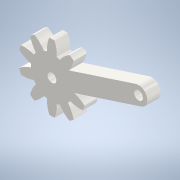
# Autodesk Inventor part: Spur Gear2
Saved by Autodesk Inventor 2021 (Build 250183000, 183)
## iProperties
CustomPartVersion: 1
Created: 2022-01-08
Part Number: Spur Gear2
Material: Steel
Document SubType Name: Modeling
Designer: Łukasz
Categories: <?xml version="1.0" encoding="UTF-16"?> <MemberInstance><Categories><FamilyTemplate><FamilyTemplateParameter ValueType="xs:double" Id="1" ObjectReferenceKey="da_z" ObjectType="kUserParameterObject"/><FamilyTemplateParameter ValueType="xs:double" Id="2" ObjectReferenceKey="da_b" ObjectType="kUserParameterObject"/><FamilyTemplateParameter ValueType="xs:double" Id="3" ObjectReferenceKey="da_beta" ObjectType="kUserParameterObject"/><FamilyTemplateParameter ValueType="xs:double" Id="4" ObjectReferenceKey="da_da" ObjectType="kUserParameterObject"/><FamilyTemplateParameter ValueType="xs:double" Id="5" ObjectReferenceKey="da_aw" ObjectType="kUserParameterObject"/><FamilyTemplateParameter ValueType="xs:string" Id="6" ObjectReferenceKey="EAIAABAAAACIAQAAAAAAAIAAAAAAAAAA" ObjectType="83910656" SubObjectId="SurfaceGeometry"/></FamilyTemplate><ParamToTemplateMap><ParamToTemplate CategoryParameter="//CategoryParameter[@InternalName='046C89C9-8512-4d59-83FE-43B91F4F132A']" TemplateParameter="1"/><ParamToTemplate CategoryParameter="//CategoryParameter[@InternalName='2552DF32-E462-4b46-AEBF-C6C7768E72AC']" TemplateParameter="2"/><ParamToTemplate CategoryParameter="//CategoryParameter[@InternalName='C9EE641D-15FC-4fae-A226-E94C4372FDD7']" TemplateParameter="3"/><ParamToTemplate><ParamToTemplate CategoryParameter="//CategoryParameter[@InternalName='00B6519A-459B-49c7-AD84-2E56D39A5744']" ConstantValue="0.035848"/></ParamToTemplate><ParamToTemplate><ParamToTemplate CategoryParameter="//CategoryParameter[@InternalName='04B31F0E-C7A6-4894-AA32-9629BEFACF47']" ConstantValue="1.000000"/></ParamToTemplate><ParamToTemplate><ParamToTemplate CategoryParameter="//CategoryParameter[@InternalName='43CBEC2E-7847-49e7-A936-2F7889FCB2D9']" ConstantValue="0.250000"/></ParamToTemplate><ParamToTemplate><ParamToTemplate CategoryParameter="//CategoryParameter[@InternalName='B1EFC894-105D-4ebd-86BF-FA20ED196853']" ConstantValue="0.302500"/></ParamToTemplate><ParamToTemplate><ParamToTemplate CategoryParameter="//CategoryParameter[@InternalName='51175063-3D10-4879-93E8-6246FE8B403D']" ConstantValue="2060000000.000000"/></ParamToTemplate><ParamToTemplate><ParamToTemplate CategoryParameter="//CategoryParameter[@InternalName='A3A52E27-4454-46a9-B0BD-C932399B70AF']" ConstantValue="0.300000"/></ParamToTemplate><ParamToTemplate><ParamToTemplate CategoryParameter="//CategoryParameter[@InternalName='91B76062-C214-41d9-B1B9-14D2AB99603D']" ConstantValue="0.250000"/></ParamToTemplate><ParamToTemplate><ParamToTemplate CategoryParameter="//CategoryParameter[@InternalName='374E806E-8B8A-4dda-A9AA-1039D6500AD2']" ConstantValue="4.000000"/></ParamToTemplate><ParamToTemplate><ParamToTemplate CategoryParameter="//CategoryParameter[@InternalName='2D373A89-B862-43d6-8D0B-0CBF12AB9F6C']" ConstantValue="0.349066"/></ParamToTemplate><ParamToTemplate CategoryParameter="//CategoryParameter[@InternalName='37777632-D6A2-4fac-9D53-DB8ACD95C989']" TemplateParameter="4"/><ParamToTemplate CategoryParameter="//CategoryParameter[@InternalName='FD1017F1-B727-4f7e-9707-0F86F1FF9423']" TemplateParameter="5"/><ParamToTemplate><ParamToTemplate CategoryParameter="//CategoryParameter[@InternalName='9E1B4470-B2D3-4ff1-B813-535BB4CDF51A']" ConstantValue="9000000.000000"/></ParamToTemplate><ParamToTemplate><ParamToTemplate CategoryParameter="//CategoryParameter[@InternalName='F8452263-BFF6-458c-9FB1-07C4B99E95CD']" ConstantValue="11400000.000000"/></ParamToTemplate><ParamToTemplate><ParamToTemplate CategoryParameter="//CategoryParameter[@InternalName='3E3BB259-FD49-497f-8171-6EBC954A3479']" ConstantValue="2.000000"/></ParamToTemplate><ParamToTemplate CategoryParameter="//CategoryParameter[@InternalName='27C3BAF2-7550-4e4b-AE2C-0DB134B7D9B7']" TemplateParameter="6"/></ParamToTemplateMap><Category DisplayName="Gear" InternalName="DC85795E-93AB-48d5-8EEE-5A27447B64BD" Mnemonic="Gear"><CategoryParameter DisplayName="z" InternalName="046C89C9-8512-4d59-83FE-43B91F4F132A" Mnemonic="z"/><CategoryParameter DisplayName="b" InternalName="2552DF32-E462-4b46-AEBF-C6C7768E72AC" Mnemonic="b"/><CategoryParameter DisplayName="||b|" InternalName="C9EE641D-15FC-4fae-A226-E94C4372FDD7" Mnemonic="beta"/><CategoryParameter DisplayName="x" InternalName="00B6519A-459B-49c7-AD84-2E56D39A5744" Mnemonic="x"/><CategoryParameter DisplayName="a*" InternalName="04B31F0E-C7A6-4894-AA32-9629BEFACF47" Mnemonic="a"/><CategoryParameter DisplayName="c*" InternalName="43CBEC2E-7847-49e7-A936-2F7889FCB2D9" Mnemonic="c"/><CategoryParameter DisplayName="r|.f|*" InternalName="B1EFC894-105D-4ebd-86BF-FA20ED196853" Mnemonic="rf"/><CategoryParameter DisplayName="E" InternalName="51175063-3D10-4879-93E8-6246FE8B403D" Mnemonic="E"/><CategoryParameter DisplayName="||m|" InternalName="A3A52E27-4454-46a9-B0BD-C932399B70AF" Mnemonic="mi"/><Category DisplayName="SpurGear" InternalName="26C5A22E-A91E-4dfd-A3B3-23CCAFAE1764" Mnemonic="SpurGear"><CategoryParameter DisplayName="m" InternalName="91B76062-C214-41d9-B1B9-14D2AB99603D" Mnemonic="m"/><CategoryParameter DisplayName="P" InternalName="374E806E-8B8A-4dda-A9AA-1039D6500AD2" Mnemonic="PP"/><CategoryParameter DisplayName="||a|" InternalName="2D373A89-B862-43d6-8D0B-0CBF12AB9F6C" Mnemonic="alpha"/><CategoryParameter DisplayName="d|.a|" InternalName="37777632-D6A2-4fac-9D53-DB8ACD95C989" Mnemonic="da"/><CategoryParameter DisplayName="a|.w|" InternalName="FD1017F1-B727-4f7e-9707-0F86F1FF9423" Mnemonic="aw"/><CategoryParameter DisplayName="||s||.Flim|" InternalName="9E1B4470-B2D3-4ff1-B813-535BB4CDF51A" Mnemonic="sFlim"/><CategoryParameter DisplayName="||s||.Hlim|" InternalName="F8452263-BFF6-458c-9FB1-07C4B99E95CD" Mnemonic="sHlim"/><CategoryParameter DisplayName="type" InternalName="3E3BB259-FD49-497f-8171-6EBC954A3479" Mnemonic="type"/><CategoryParameter DisplayName="PitchDiameter" InternalName="27C3BAF2-7550-4e4b-AE2C-0DB134B7D9B7" Mnemonic="IDS_PITCHDIAM"/></Category></Category></Categories></MemberInstance>
Density: 1 g/cm^3
Appearance: Steel
Author: Łukasz
Autodesk Inventor part; units mm, degrees
ref_plane "YZ Plane" through (0, 0, 0) normal (1, 0, 0) x (0, 1, 0)
ref_plane "XZ Plane" through (0, 0, 0) normal (0, 1, 0) x (-1, 0, 0)
ref_plane "XY Plane" through (0, 0, 0) normal (0, 0, 1) x (1, 0, 0)
sketch "Sketch1" plane through (0, 0, 0) normal (0, 0, 1) x (1, 0, 0)
  circle A0 centre (0, 0) radius 15.0851
  dimension "d0" = 30.1702
  constraints: 1 centre point
  measures "d0" diameter of A0
extrude "Extrusion1" add sketch "Sketch1" along normal blind 6
ref_plane "Work Plane2" through (0, 0, 3) normal (0, 0, 1) x (-1, 0, 0)
sketch "Sketch2" plane through (0, 0, 0) normal (0, 0, -1) x (-1, 0, 0)
  circle A0 centre (0, 0) radius 15.0851 projected
  circle A1 centre (0, 0) radius 12.5
  dimension "d3" = 25
  constraints: 1 centre point, 1 coincident
  measures "d3" diameter of A1
surface extrude "Pitch Diameter" sketch "Sketch2" against normal through all shown no curves A1
ref_plane "Work Plane8" through (0, 0, 0) normal (0.9510565, 0.309017, 0) x (0, 0, 1)
ref_plane "Work Plane9" through (0, 0, 0) normal (1, 0, 0) x (0, 1, 0)
spur gear teeth "Spur Gear" teeth 10 pitch diameter 25 tip diameter 30.1702 root diameter 18.9292 face width 6 start plane through (0, 0, 0) normal (0, 0, -1) x (-1, 0, 0)
sketch "Sketch3" plane through (0, 0, 0) normal (0, 0, -1) x (-1, 0, 0)
  circle A0 centre (0, 0) radius 2
  dimension "d49" = 4
  constraints: 1 centre point, 1 coincident
  measures "d49" diameter of A0
extrude "Extrusion2" cut sketch "Sketch3" against normal up to surface (6 mm away)
sketch "Sketch4" plane through (0, 0, 0) normal (0, 0, -1) x (-1, 0, 0)
  circle A0 centre (-31.2139, 36.6123) radius 2 projected
  line L0 (-4.8178, 32.2415) -> (-29.9778, 40.4165) projected
  arc A1 (-29.9778, 40.4165) -> (-32.45, 32.8081) centre (-31.2139, 36.6123) ccw projected
  line L1 (-32.45, 32.8081) -> (-7.2899, 24.6331) projected
  arc A2 (-7.2899, 24.6331) -> (-7.2592, 22.759) centre (7.7794, 23.9426) ccw projected
  arc A3 (-7.2592, 22.759) -> (-1.4237, 21.7331) centre (-2.0301, 35.3932) ccw projected
  arc A4 (-1.4237, 21.7331) -> (-0.9647, 20.3206) centre (7.7794, 23.9426) ccw projected
  arc A5 (-0.9647, 20.3206) -> (-5.0828, 16.0606) centre (6.5738, 8.913) ccw projected
  arc A6 (-5.0828, 16.0606) -> (-3.6914, 14.1456) centre (7.7794, 23.9426) ccw projected
  arc A7 (-3.6914, 14.1456) -> (1.6326, 16.7456) centre (-6.8872, 27.4404) ccw projected
  arc A8 (1.6326, 16.7456) -> (2.8342, 15.8727) centre (7.7794, 23.9426) ccw projected
  arc A9 (2.8342, 15.8727) -> (2.0066, 10.0058) centre (15.6383, 11.0747) ccw projected
  arc A10 (2.0066, 10.0058) -> (4.2579, 9.2743) centre (7.7794, 23.9426) ccw projected
  arc A11 (4.2579, 9.2743) -> (7.0368, 14.5072) centre (-6.1421, 18.1516) ccw projected
  arc A12 (7.0368, 14.5072) -> (8.522, 14.5072) centre (7.7794, 23.9426) ccw projected
  arc A13 (8.522, 14.5072) -> (11.301, 9.2743) centre (21.7009, 18.1516) ccw projected
  arc A14 (11.301, 9.2743) -> (13.5522, 10.0058) centre (7.7794, 23.9426) ccw projected
  arc A15 (13.5522, 10.0058) -> (12.7247, 15.8727) centre (-0.0794, 11.0747) ccw projected
  arc A16 (12.7247, 15.8727) -> (13.9262, 16.7456) centre (7.7794, 23.9426) ccw projected
  arc A17 (13.9262, 16.7456) -> (19.2502, 14.1456) centre (22.446, 27.4404) ccw projected
  arc A18 (19.2502, 14.1456) -> (20.6416, 16.0606) centre (7.7794, 23.9426) ccw projected
  arc A19 (20.6416, 16.0606) -> (16.5236, 20.3206) centre (8.985, 8.913) ccw projected
  arc A20 (16.5236, 20.3206) -> (16.9825, 21.7331) centre (7.7794, 23.9426) ccw projected
  arc A21 (16.9825, 21.7331) -> (22.818, 22.759) centre (17.589, 35.3932) ccw projected
  arc A22 (22.818, 22.759) -> (22.818, 25.1262) centre (7.7794, 23.9426) ccw projected
  arc A23 (22.818, 25.1262) -> (16.9825, 26.1521) centre (17.589, 12.492) ccw projected
  arc A24 (16.9825, 26.1521) -> (16.5236, 27.5646) centre (7.7794, 23.9426) ccw projected
  arc A25 (16.5236, 27.5646) -> (20.6416, 31.8246) centre (8.985, 38.9722) ccw projected
  arc A26 (20.6416, 31.8246) -> (19.2502, 33.7396) centre (7.7794, 23.9426) ccw projected
  arc A27 (19.2502, 33.7396) -> (13.9262, 31.1396) centre (22.446, 20.4448) ccw projected
  arc A28 (13.9262, 31.1396) -> (12.7247, 32.0125) centre (7.7794, 23.9426) ccw projected
  arc A29 (12.7247, 32.0125) -> (13.5522, 37.8794) centre (-0.0794, 36.8105) ccw projected
  arc A30 (13.5522, 37.8794) -> (11.301, 38.6109) centre (7.7794, 23.9426) ccw projected
  arc A31 (11.301, 38.6109) -> (8.522, 33.378) centre (21.7009, 29.7336) ccw projected
  arc A32 (8.522, 33.378) -> (7.0368, 33.378) centre (7.7794, 23.9426) ccw projected
  arc A33 (7.0368, 33.378) -> (4.2579, 38.6109) centre (-6.1421, 29.7336) ccw projected
  arc A34 (4.2579, 38.6109) -> (2.0066, 37.8794) centre (7.7794, 23.9426) ccw projected
  arc A35 (2.0066, 37.8794) -> (2.8342, 32.0125) centre (15.6383, 36.8105) ccw projected
  arc A36 (2.8342, 32.0125) -> (1.6326, 31.1396) centre (7.7794, 23.9426) ccw projected
  arc A37 (1.6326, 31.1396) -> (-3.6914, 33.7396) centre (-6.8872, 20.4448) ccw projected
  arc A38 (-3.6914, 33.7396) -> (-4.8178, 32.2415) centre (7.7794, 23.9426) ccw projected
  circle A39 centre (7.7794, 23.9426) radius 1.5 projected
  line L2 (-1.2361, -3.8042) -> (-40.2294, 8.8655)
  line L3 (-42.7975, 13.9058) -> (-42.7975, 13.9058)
  line L4 (-37.7572, 16.4739) -> (1.2361, 3.8042)
  line L5 (1.2361, 3.8042) -> (-1.2361, -3.8042)
  circle A40 centre (-38.9933, 12.6697) radius 2
  arc A41 (-42.7975, 13.9058) -> (-40.2294, 8.8655) centre (-38.9933, 12.6697) ccw
  arc A42 (-37.7572, 16.4739) -> (-42.7975, 13.9058) centre (-38.9933, 12.6697) ccw
  line L6 (-11.3742, 7.9016) -> (-13.8464, 0.2931)
  circle A43 centre (0, 0) radius 2 projected
  point P0 (0, 0)
  point P1 (-41.5615, 17.71)
  point P2 (-44.0336, 10.1015)
  point P3 (-42.7975, 13.9058)
  point P4 (-0.618, -1.9021)
  point P5 (0.618, 1.9021)
  dimension "d61" = 45
  dimension "d62" = 8
  dimension "d63" = 4
  dimension "d64" = 0
  dimension "d65" = 4
  dimension "d66" = 4
  dimension "d67" = 4
  dimension "d68" = 0
  constraints: 10 end point, 6 point on line, 4 point on circle, 4 tangent, 3 centre point, 2 parallel, 2 perpendicular, 1 concentric
  measures "d61" distance of point (-41.561, 17.71) L4.end
  measures "d62" distance of point (-44.034, 10.102) point (-41.561, 17.71)
  measures "d63" distance from line of point (0, 0) L2
  measures "d64" distance from line of point (0, 0) L5
  measures "d65" diameter of A40
  measures "d66" distance from line of L3 A40.centre
  measures "d67" radius of A41
  measures "d68" distance of A43.centre point (0, 0)
extrude "Extrusion3" add sketch "Sketch4" against normal up to surface (6 mm away) contours L2 L6 L4 L5 A43 | L2 A41 A42 L4 L6
equation "\"d0\" = da_da"
equation "\"d1\" = da_b"
equation "\"d3\" = da_d"
equation "\"d16\" = da_aw"
equation "\"d43\" = da_aw"
equation "\"d46\" = da_aw"
equation "\"da_da\" = 30.170238"
equation "\"da_b\" = 6"
equation "\"da_d\" = 25"
equation "\"da_aw\" = 25.174739"
body "Solid1"
body "Srf1"
